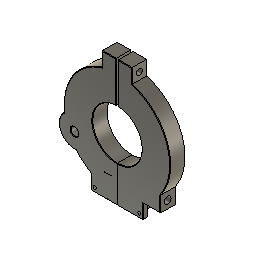
Tiefenstop (Autodesk Fusion 360 design; units mm, degrees)
Autodesk Fusion 360 part; units mm, degrees
sketch "Sketch1" plane through (0, 0, 0) normal (0, 1, 0) x (1, 0, 0)
  circle A0 centre (0, 0) radius 20
  circle A1 centre (0, 0) radius 43
  line L0 (-12, -41.2916) -> (-12, -53)
  line L1 (-12, -53) -> (12, -53)
  line L2 (12, -53) -> (12, -41.2916)
  line L3 (0, -53) -> (0, 0) construction
  line L4 (-1, -19.975) -> (-1, -53)
  line L5 (1, -19.975) -> (1, -53)
  line L6 (-21, 37.5233) -> (-21, 49)
  line L7 (-21, 49) -> (21, 49)
  line L8 (21, 49) -> (21, 37.5233)
  line L9 (0, 49) -> (0, 0) construction
  circle A2 centre (-18, 46) radius 1.2
  circle A3 centre (18, 46) radius 1.2
  line L10 (18, 46) -> (-18, 46) construction
  circle A4 centre (-34.5, 15) radius 12.5
  line L11 (-34.5, 15) -> (-34.5, 0)
  line L12 (-34.5, 0) -> (43, 0)
  line L13 (-37.4445, 20.1) -> (-40.389, 15)
  line L14 (-40.389, 15) -> (-37.4445, 9.9)
  line L15 (-37.4445, 9.9) -> (-31.5555, 9.9)
  line L16 (-31.5555, 9.9) -> (-28.611, 15)
  line L17 (-28.611, 15) -> (-31.5555, 20.1)
  line L18 (-31.5555, 20.1) -> (-37.4445, 20.1)
  circle A5 centre (-34.5, 15) radius 3.2
  line L19 (35, 24.98) -> (35, 37.5233)
  line L20 (35, 37.5233) -> (21, 37.5233)
  point P0 (0, 46)
  point P1 (-34.5, 15)
  dimension "d1" = 40
  dimension "d2" = 86
  dimension "d3" = 53
  dimension "d4" = 24
  dimension "d5" = 2
  dimension "d6" = 36
  dimension "d7" = 2.4
  dimension "d8" = 3
  dimension "d9" = 3
  dimension "d10" = 46
  dimension "d11" = 15
  dimension "d13" = 10.2
  dimension "d14" = 25
  dimension "d15" = 6.4
  dimension "d45" = 8.5
  dimension "d46" = 35
  constraint coincident A0.centre A1.centre
  constraint coincident A1 L0.start
  constraint vertical L0
  constraint perpendicular L0 L1
  constraint coincident A1 L2.end
  constraint perpendicular L1 L2
  constraint midpoint L1 L3.start
  constraint vertical L3
  constraint coincident A0 L4.start
  constraint coincident L1 L4.end
  constraint perpendicular L1 L4
  constraint coincident A0 L5.start
  constraint coincident L1 L5.end
  constraint perpendicular L1 L5
  constraint equal L4 L5
  constraint coincident A1 L6.start
  constraint vertical L6
  constraint perpendicular L6 L7
  constraint coincident A1 L8.end
  constraint perpendicular L7 L8
  constraint midpoint L7 L9.start
  constraint vertical L9
  constraint coincident A3.centre L10.start
  constraint coincident A2.centre L10.end
  constraint horizontal L10
  constraint midpoint L10 P0
  constraint coincident L9 P0
  constraint equal A2 A3
  constraint coincident P1 A4.centre
  constraint vertical L11
  constraint coincident A1 L12.end
  constraint perpendicular L11 L12
  constraint horizontal A0.centre L11.end
  constraint horizontal L15
  constraint coincident A1 L19.start
  constraint vertical L19
  constraint horizontal L20
  measures "d1" diameter of A0
  measures "d2" diameter of A1
  measures "d3" distance of L3.start A0.centre
  measures "d4" distance of L0.end L1.end
  measures "d5" distance of L4 L5
  measures "d6" distance of A3.centre A2.centre
  measures "d7" diameter of A2
  measures "d8" distance of L7 L10
  measures "d9" distance of L6 A2.centre
  measures "d10" distance of A0.centre L10
  measures "d11" vertical distance of A0.centre A4.centre
  measures "d13" distance of L15 L18
  measures "d14" diameter of A4
  measures "d15" diameter of A5
  measures "d45" distance of A1 L11.end
  measures "d46" horizontal distance of P0 L19.end
extrude "Extrude1" add sketch "Sketch1" along normal blind 12 contours A0 A1 L4 A4 L11 L12 | A0 A1 L5 L12 | A0 A1 A4 L11 L12 | A1 L0 L1 L4 | A1 L1 L2 L5 | A1 A4 L11 L13 L15 L16 L17 L18 | A1 A4 L11 L14 L15 | A1 A4 L13 L14 | A1 L19 L20 | A1 L13 L14 makes body 1
extrude "Extrude2" add sketch "Sketch1" along normal blind 5 contours A1 L13 L14 L15 L16 L17 L18 bodies 1
extrude "Extrude3" add sketch "Sketch1" along normal blind 3.4 contours A1 L6 L7 L8 bodies 1
sketch "Sketch2" plane through (0, 0, 0) normal (1, 0, 0) x (0, 1, 0)
  circle A0 centre (16.5, -51) radius 2.4
  line L0 (12, -43) -> (18.7736, -46.2255)
  arc A1 (14.2264, -55.7745) -> (18.7736, -46.2255) centre (16.5, -51) ccw
  line L1 (14.2264, -55.7745) -> (0, -49)
  line L2 (12, -43) -> (12, -37.4069)
  line L3 (0, -37.4069) -> (0, -49)
  line L4 (0, -37.4069) -> (12, -37.4069)
  line L5 (12, -5.5176) -> (12, 41.2916)
  point P0 (3.4, -49)
  point P1 (0, -49)
  dimension "d22" = 4.5
  dimension "d23" = 8
  dimension "d24" = 4.8
  constraint coincident A0.centre A1.centre
  constraint coincident L0.end A1.end
  constraint tangent L0 A1
  constraint coincident P1 L1.end
  constraint tangent A1 L1
  constraint parallel L0 L1
  measures "d22" horizontal distance of A0.centre L0.start
  measures "d23" vertical distance of A0.centre L0.start
  measures "d24" diameter of A0
extrude "Extrude4" add sketch "Sketch2" along normal mid plane 16 bodies 1
chamfer "Chamfer1" distance 7 distance2 0.7 1 edges at (0, 12, -43) measured on face at (2.6667, 16.5157, -45.1503) on bodies 1
sketch "Sketch3" plane through (35, 0, 0) normal (1, 0, 0) x (0, -1, 0)
  line L0 (0, -37.5233) -> (0, -24.98)
  line L1 (-12, -24.98) -> (-12, -37.5233)
  line L2 (-6, 24.98) -> (-6, 37.5233) construction
  circle A0 centre (-6, 31.2517) radius 2.8
  line L3 (-8.9445, 26.1517) -> (-3.0555, 26.1517)
  line L4 (-3.0555, 26.1517) -> (-0.111, 31.2517)
  line L5 (-0.111, 31.2517) -> (-3.0555, 36.3517)
  line L6 (-3.0555, 36.3517) -> (-8.9445, 36.3517)
  line L7 (-8.9445, 36.3517) -> (-11.889, 31.2517)
  line L8 (-11.889, 31.2517) -> (-8.9445, 26.1517)
  line L9 (0, 24.98) -> (0, 37.5233)
  line L10 (0, 37.5233) -> (-12, 37.5233)
  line L11 (-12, 37.5233) -> (-12, 24.98)
  line L12 (-12, 24.98) -> (0, 24.98)
  line L13 (-8.9445, 26.1517) -> (-12, 26.1517)
  line L14 (-8.9445, 36.3517) -> (-12, 36.3517)
  point P0 (-6, 31.2517)
  dimension "d30" = 5.6
  dimension "d31" = 10.2
  constraint coincident L2 P0
  constraint midpoint L2 P0
  constraint coincident P0 A0.centre
  constraint midpoint L2.end L10
  constraint midpoint L2.start L12
  constraint coincident L8 L3.start
  constraint coincident L3.start L8.end
  constraint horizontal L3
  constraint coincident L11 L13.end
  constraint perpendicular L11 L13
  constraint coincident L11 L14.end
  constraint perpendicular L11 L14
  measures "d30" diameter of A0
  measures "d31" distance of L5 L8
extrude "Extrude5" cut sketch "Sketch3" against normal blind 50 contours A0 bodies 1
extrude "Extrude6" cut sketch "Sketch3" against normal blind 5.2 from surface at -40 contours L3 L4 L5 L6 L7 L8 | L7 L8 L11 L13 L14 bodies 1
sketch "Sketch4" plane through (-12, 0, 0) normal (-1, 0, 0) x (0, -1, 0)
  line L0 (0, 41.2916) -> (0, 53)
  line L1 (0, 53) -> (-12, 53)
  line L2 (-12, 53) -> (-12, 41.2916)
  line L3 (-12, 41.2916) -> (0, 41.2916)
  line L4 (-12, 47.1458) -> (0, 47.1458) construction
  circle A0 centre (-6, 47.1458) radius 2.4
  line L5 (-2.25, 49.3109) -> (-6, 51.4759)
  line L6 (-6, 51.4759) -> (-9.75, 49.3109)
  line L7 (-9.75, 49.3109) -> (-9.75, 44.9808)
  line L8 (-9.75, 44.9808) -> (-6, 42.8157)
  line L9 (-6, 42.8157) -> (-2.25, 44.9808)
  line L10 (-2.25, 44.9808) -> (-2.25, 49.3109)
  point P0 (-6, 47.1458)
  dimension "d39" = 4.8
  dimension "d40" = 7.5
  constraint midpoint L2 L4.start
  constraint midpoint L0 L4.end
  constraint midpoint L4 P0
  constraint coincident P0 A0.centre
  constraint vertical L10
  measures "d39" diameter of A0
  measures "d40" distance of L7 L10
extrude "Extrude7" cut sketch "Sketch4" against normal blind 3 contours L5 L6 L7 L8 L9 L10 bodies 1
extrude "Extrude8" cut 1 faces at (-12, 6.178, 47.8553) along direction (1, 0, 0) blind 44 on bodies 1 bodies 1
chamfer "Chamfer2" distance 0.4 angle 45 16 edges at (40.6231, 0, 14.0985) (-27.5272, 0, -33.0341) (-45.9634, 0, -19.9841) (-35.9761, 0, 23.5525) (21, 0, -43.2617) (-21, 0, -43.2617) (-12, 0, 47.1458) (-6.5, 0, 53) (0, 0, -20) (-1, 0, 36.4875) (1, 0, 36.4875) (6.5, 0, 53) (12, 0, 47.1458) (-37.4834, 0, -16.1572) (35, 0, -31.2517) (28, 0, -37.5233) on bodies 1
split "Split1" by plane through (0, 0, 0) normal (1, 0, 0) bodies 1 makes body 2 at (22.943, 0, -25.718)
